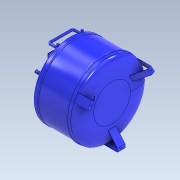
# Autodesk Inventor part: estanque
Saved by Autodesk Inventor 2022 (Build 260153000, 153)
## iProperties
Created: 2022-11-16
Part Number: estanque
Material: Generic
Document SubType Name: Modeling
Designer: ferna
Density: 1 g/cm^3
Appearance: Blue - Wall Paint - Glossy
Author: ferna
Autodesk Inventor part; units mm, degrees
ref_plane "YZ Plane" through (0, 0, 0) normal (1, 0, 0) x (0, 1, 0)
ref_plane "XY Plane" through (0, 0, 0) normal (0, 0, 1) x (1, 0, 0)
sketch "Sketch1" plane through (0, 0, 0) normal (0, 1, 0) x (-1, 0, 0)
  line L0 (0, 0) -> (0, -200)
  line L1 (0, -200) -> (150, -200)
  arc A0 (150, -200) -> (158, -200) centre (154, -197) ccw
  arc A1 (-8, -199.9777) -> (0, -200) centre (-4, -200) ccw
  line L2 (158, -200) -> (173, -200)
  line L3 (-8, -200) -> (-23, -200)
  ellipse E0 centre (173, -100) end of major axis (197.5923, -100) minor radius 100
  line L4 (197.5923, -100) -> (197.5923, 0)
  ellipse E1 centre (-25, -100) end of major axis (-0.4078, -100) minor radius 100
  line L5 (-0.4078, -100) -> (-0.4078, 0)
  line L6 (-49.5923, -100) -> (-49.5923, 0)
  line L7 (-49.5923, 0) -> (197.5923, 0)
  line L8 (-23, -200) -> (-25, -200)
  line L9 (-25, 0) -> (-0.4078, 0)
  point P0 (-25, -200)
  dimension "d0" = 200
  dimension "d1" = 150
  dimension "d2" = 8
  dimension "d3" = 5
  dimension "d4" = 8
  dimension "d5" = 15
  dimension "d6" = 15
  constraints: 20 end point, 7 vertical, 5 horizontal, 5 point on circle, 2 centre point, 1 collinear, 1 perpendicular, 1 point on line, 1 tangent, 10 other
  measures "d0" distance of L0.start L0.end
  measures "d1" distance of L0.end L1.end
  measures "d2" distance of L1.end L2.start
  measures "d3" radius of A0
  measures "d4" distance of L0.end A1.start
  measures "d5" distance of L2.start L2.end
  measures "d6" distance of L3.start L3.end
revolve "Revolution1" add sketch "Sketch1" angle 360 about axis through (49.5923, 0, 0) along (-1, 0, 0)
sketch "Sketch2" plane through (-197.5923, 0, 0) normal (-1, 0, 0) x (0, 0, 1)
  point P0 (0, 0)
ref_plane "Work Plane2" through (0, 189.25, 0) normal (0, 1, 0) x (-1, 0, 0)
sketch "Sketch3" plane through (0, 189.25, 0) normal (0, 1, 0) x (-1, 0, 0)
  circle A0 centre (183.8309, 60.3098) radius 6.2779
  point P0 (0, 0)
  constraints: 1 centre point
sketch3d "3D Sketch1"
  line L0 (-183.8309, 189.25, 60.3098) -> (-183.8309, 179.25, 60.3098)
  arc A0 (-183.8309, 179.25, 60.3098) -> (-193.8309, 169.25, 60.3098) centre (-193.8309, 179.25, 60.3098) ccw
  line L1 (-193.8309, 169.25, 60.3098) -> (-223.8309, 169.25, 60.3098)
  arc A1 (-223.8309, 169.25, 60.3098) -> (-233.8309, 169.25, 50.3098) centre (-223.8309, 169.25, 50.3098) ccw
  line L2 (-233.8309, 169.25, 50.3098) -> (-233.8309, 169.25, -60.7848)
  arc A2 (-233.8309, 169.25, -60.7848) -> (-223.8309, 169.25, -70.7848) centre (-223.8309, 169.25, -60.7848) ccw
  line L3 (-223.8309, 169.25, -70.7848) -> (-193.8309, 169.25, -70.7848)
  arc A3 (-193.8309, 169.25, -70.7848) -> (-183.8309, 179.25, -70.7848) centre (-193.8309, 179.25, -70.7848) ccw
  line L4 (-183.8309, 179.25, -70.7848) -> (-183.8309, 189.25, -70.7848)
  dimension "d9" = 20
  dimension "d10" = 50
  dimension "d11" = 50
  dimension "d12" = 20
  dimension "d13" = 10
  dimension "d14" = 10
  dimension "d15" = 10
  dimension "d16" = 10
sweep "Sweep1" add profiles "Sketch3" path "3D Sketch1"
mirror "Mirror1" about plane through (0, 0, 0) normal (0, 1, 0) of "Sweep1"
ref_plane "Work Plane3" through (99.5923, 0, 0) normal (1, 0, 0) x (0, 0, -1)
sketch "Sketch4" plane through (99.5923, 0, 0) normal (1, 0, 0) x (0, 0, -1)
  circle A0 centre (0, 0) radius 200 projected
  line L0 (21.7689, -198.8118) -> (-20.4699, -198.8118)
  line L1 (-20.4699, -198.8118) -> (-20.4699, -195.5552)
  line L2 (-20.4699, -195.5552) -> (21.7689, -195.5552)
  line L3 (21.7689, -195.5552) -> (21.7689, -198.8118)
  circle A1 centre (0, 0) radius 200 projected
  line L4 (161.2916, 118.2583) -> (182.411, 81.6785)
  line L5 (158.4713, 116.63) -> (161.2916, 118.2583)
  line L6 (179.5907, 80.0502) -> (158.4713, 116.63)
  line L7 (182.411, 81.6785) -> (179.5907, 80.0502)
  line L8 (-183.0605, 80.5534) -> (-161.9411, 117.1333)
  line L9 (-180.2402, 78.9251) -> (-183.0605, 80.5534)
  line L10 (-159.1208, 115.505) -> (-180.2402, 78.9251)
  line L11 (-161.9411, 117.1333) -> (-159.1208, 115.505)
  point P0 (0, 0)
  point P1 (200, 0)
  dimension "d22" = 360
  constraints: 24 end point, 2 parallel, 1 horizontal, 1 perpendicular, 1 point on circle, 25 other
extrude "Extrusion1" add sketch "Sketch4" against normal up to next contours L4 L7 L6 L5 | L8 L11 L10 L9 | L0 L1 L2 L3
sketch "Sketch6" plane through (25, 118.2583, -161.2916) normal (0, 0.8660254, 0.5) x (1, 0, 0)
  line L0 (74.5923, -3.0263) -> (72.0923, -3.0263)
  line L1 (72.0923, -3.0263) -> (72.0923, -18.0263)
  line L2 (72.0923, -18.0263) -> (74.5923, -18.0263)
  line L3 (74.5923, -18.0263) -> (74.5923, -3.0263)
  line L4 (74.5923, -18.0263) -> (-2.5422, -109.9517)
  line L5 (74.5923, -18.0263) -> (194.5923, -18.0263) construction
  line L6 (72.0923, -18.0263) -> (-5.0422, -109.9517)
  line L7 (72.0923, -18.0263) -> (192.0923, -18.0263) construction
  line L8 (-17, -398.8118) -> (-17, 1.1882) projected
  line L9 (-5.0422, -109.9517) -> (-2.5422, -109.9517)
  point P0 (-25, -198.8118)
  dimension "d26" = 2.5
  dimension "d27" = 15
  dimension "d28" = 120
  dimension "d29" = 130
  dimension "d30" = 120
  dimension "d31" = 130
  constraints: 18 end point, 3 horizontal, 2 equal length, 2 parallel, 1 perpendicular
  measures "d26" distance of L2.end L1.end
  measures "d27" distance of L1.end L0.end
  measures "d28" distance of L2.end L4.end
  measures "d29" angle of L4 L5
  measures "d30" distance of L1.end L6.end
  measures "d31" angle of L6 L7
extrude "Extrusion2" add sketch "Sketch6" against normal up to surface (42.2388 mm away)
sketch "Sketch7" plane through (99.5923, -198.8118, 20.4699) normal (0, 0, 1) x (1, 0, 0)
  line L0 (0, 0) -> (0, 3.2566) projected
  line L1 (0, 3.2566) -> (-2.5, 3.2566)
  line L2 (-2.5, 3.2566) -> (-2.5, 18.2566)
  line L3 (-2.5, 18.2566) -> (0, 18.2566)
  line L4 (0, 18.2566) -> (0, 3.2566)
  line L5 (0, 18.2566) -> (-77.1345, 110.1819)
  line L6 (0, 18.2566) -> (120, 18.2566) construction
  line L7 (-2.5, 18.2566) -> (-79.6345, 110.1819)
  line L8 (-2.5, 18.2566) -> (117.5, 18.2566) construction
  line L9 (-79.6345, 110.1819) -> (-77.1345, 110.1819)
  point P0 (-99.5923, 198.8118)
  dimension "d34" = 2.5
  dimension "d35" = 15
  dimension "d36" = 120
  dimension "d37" = 130
  dimension "d38" = 120
  dimension "d39" = 130
  constraints: 18 end point, 3 horizontal, 2 equal length, 2 parallel, 1 perpendicular
  measures "d34" distance of L2.end L3.end
  measures "d35" distance of L1.end L2.end
  measures "d36" distance of L3.end L5.end
  measures "d37" angle of L6 L5
  measures "d38" distance of L2.end L7.end
  measures "d39" angle of L8 L7
extrude "Extrusion3" add sketch "Sketch7" against normal up to surface (42.2388 mm away)
sketch "Sketch8" plane through (25, 80.5534, 183.0605) normal (0, -0.8660254, 0.5) x (1, 0, 0)
  line L0 (74.5923, 0) -> (74.5923, -3.2566) projected
  line L1 (74.5923, -3.2566) -> (72.0923, -3.2566)
  line L2 (72.0923, -3.2566) -> (72.0923, -18.2566)
  line L3 (72.0923, -18.2566) -> (74.5923, -18.2566)
  line L4 (74.5923, -18.2566) -> (74.5923, -3.2566)
  line L5 (74.5923, -18.2566) -> (-2.5422, -110.1819)
  line L6 (74.5923, -18.2566) -> (194.5923, -18.2566) construction
  line L7 (72.0923, -18.2566) -> (-5.0422, -110.1819)
  line L8 (72.0923, -18.2566) -> (192.0923, -18.2566) construction
  line L9 (-25, -398.8118) -> (-25, 1.1882) projected
  line L10 (-5.0422, -110.1819) -> (-2.5422, -110.1819)
  point P0 (-25, -198.8118)
  dimension "d42" = 2.5
  dimension "d43" = 15
  dimension "d44" = 120
  dimension "d45" = 130
  dimension "d46" = 120
  dimension "d47" = 130
  constraints: 18 end point, 3 horizontal, 2 equal length, 2 parallel, 1 perpendicular
  measures "d42" distance of L3.end L2.end
  measures "d43" distance of L2.end L1.end
  measures "d44" distance of L3.end L5.end
  measures "d45" angle of L5 L6
  measures "d46" distance of L2.end L7.end
  measures "d47" angle of L7 L8
extrude "Extrusion4" add sketch "Sketch8" against normal up to surface (42.2388 mm away)
sketch "Sketch9" plane through (99.5923, 0, 0) normal (1, 0, 0) x (0, 0, -1)
  line L0 (-20.4699, -198.8118) -> (21.7689, -198.8118) projected
  line L1 (21.7689, -198.8118) -> (0.6494, -198.8118)
  line L2 (0.6494, -198.8118) -> (0.6494, -189.6833)
  circle A0 centre (0.6494, -189.6833) radius 2.5
  circle A1 centre (163.9458, 95.404) radius 2.5
  circle A2 centre (-164.5952, 94.2792) radius 2.5
  point P0 (0, 0)
  point P1 (0, 0)
  point P2 (0, 0)
  dimension "d50" = 21.1195
  dimension "d51" = 9.1285
  dimension "d52" = 5
  dimension "d55" = 360
  constraints: 4 end point, 3 centre point, 3 coincident, 1 perpendicular, 1 point on line, 8 other
  measures "d50" distance of L0.end L1.end
  measures "d51" distance of L1.end L2.end
  measures "d52" diameter of A0
extrude "Extrusion5" cut sketch "Sketch9" against normal blind 10
sketch "Sketch10" plane through (-197.5923, 0, 0) normal (-1, 0, 0) x (0, 0, 1)
  line L0 (125.5067, 66.7791) -> (-125.5067, 66.7791)
  line L1 (-125.5067, 66.7791) -> (-125.5067, -66.7791)
  line L2 (-125.5067, -66.7791) -> (125.5067, -66.7791)
  line L3 (125.5067, -66.7791) -> (125.5067, 66.7791)
  line L4 (125.5067, 66.7791) -> (-125.5067, -66.7791) construction
  line L5 (-125.5067, 66.7791) -> (125.5067, -66.7791) construction
  circle A0 centre (125.5067, 66.7791) radius 8
  circle A1 centre (125.5067, -66.7791) radius 8
  circle A2 centre (-125.5067, 66.7791) radius 8
  circle A3 centre (-125.5067, -66.7791) radius 8
  line L6 (-60.3098, 136.1742) -> (60.3098, 136.1742)
  line L7 (60.3098, 136.1742) -> (60.3098, -136.1742)
  line L8 (60.3098, -136.1742) -> (-60.3098, -136.1742)
  line L9 (-60.3098, -136.1742) -> (-60.3098, 136.1742)
  line L10 (-60.3098, 136.1742) -> (60.3098, -136.1742) construction
  line L11 (60.3098, 136.1742) -> (-60.3098, -136.1742) construction
  line L12 (-60.3098, 88.4499) -> (60.3098, 88.4499)
  line L13 (60.3098, 88.4499) -> (60.3098, -88.4499)
  line L14 (60.3098, -88.4499) -> (-60.3098, -88.4499)
  line L15 (-60.3098, -88.4499) -> (-60.3098, 88.4499)
  line L16 (-60.3098, 88.4499) -> (60.3098, -88.4499) construction
  line L17 (60.3098, 88.4499) -> (-60.3098, -88.4499) construction
  line L18 (-60.3098, 93.5116) -> (60.3098, 93.5116)
  line L19 (60.3098, 93.5116) -> (60.3098, -93.5116)
  line L20 (60.3098, -93.5116) -> (-60.3098, -93.5116)
  line L21 (-60.3098, -93.5116) -> (-60.3098, 93.5116)
  circle A4 centre (0, 0) radius 100 projected
  line L22 (-60.3098, 93.5116) -> (60.3098, -93.5116) construction
  line L23 (60.3098, 93.5116) -> (-60.3098, -93.5116) construction
  line L24 (-60.3098, 90.6457) -> (60.3098, 90.6457)
  line L25 (60.3098, 90.6457) -> (60.3098, -90.6457)
  line L26 (60.3098, -90.6457) -> (-60.3098, -90.6457)
  line L27 (-60.3098, -90.6457) -> (-60.3098, 90.6457)
  line L28 (-60.3098, 90.6457) -> (60.3098, -90.6457) construction
  line L29 (60.3098, 90.6457) -> (-60.3098, -90.6457) construction
  point P0 (0, 0)
  point P1 (-100, 0)
  dimension "d22" = 360
  dimension "d59" = 16
  dimension "d60" = 16
  dimension "d61" = 16
  dimension "d62" = 16
  constraints: 60 end point, 10 midpoint, 10 parallel, 5 horizontal, 5 perpendicular, 4 centre point, 4 coincident, 3 point on line, 1 horizontal alignment
  measures "d59" diameter of A0
  measures "d60" diameter of A1
  measures "d61" diameter of A2
  measures "d62" diameter of A3
extrude "Extrusion6" add sketch "Sketch10" along normal blind 40 and the other way blind 25.375 contours A2 L1 L0 | L0 L1 A2 | A3 L2 L1 | L1 L2 A3 | L9 L24 A4 L12 | A4 L24 L12 | A4 L24 L7 L12 | L14 A4 L26 L9 | L14 A4 L26 | A0 L3 L0 | L0 L3 A0 | L14 L7 L26 A4 | A1 L3 L2 | L2 L3 A1
sketch "Sketch11" plane through (-237.5923, 0, 0) normal (-1, 0, 0) x (0, 0, 1)
  line L0 (-60.3098, 88.4499) -> (60.3098, 88.4499)
  line L1 (60.3098, 88.4499) -> (60.3098, 118.4499)
  line L2 (60.3098, 118.4499) -> (-60.3098, 118.4499)
  line L3 (-60.3098, 118.4499) -> (-60.3098, 88.4499)
  line L4 (60.3098, -88.4499) -> (-60.3098, -88.4499) projected
  line L5 (-60.3098, -88.4499) -> (60.3098, -88.4499)
  line L6 (60.3098, -88.4499) -> (60.3098, -118.4499)
  line L7 (60.3098, -118.4499) -> (-60.3098, -118.4499)
  line L8 (-60.3098, -118.4499) -> (-60.3098, -88.4499)
  line L9 (-50, -105) -> (50, -105)
  line L10 (50, -105) -> (50, 105)
  line L11 (50, 105) -> (-50, 105)
  line L12 (-50, 105) -> (-50, -105)
  line L13 (-50, -105) -> (50, 105) construction
  line L14 (50, -105) -> (-50, 105) construction
  circle A0 centre (-50, 105) radius 5
  circle A1 centre (50, 105) radius 5
  circle A2 centre (-50, -105) radius 5
  circle A3 centre (50, -105) radius 5
  point P0 (0, 0)
  dimension "d67" = 30
  dimension "d68" = 30
  dimension "d69" = 100
  dimension "d70" = 210
  dimension "d71" = 10
  dimension "d72" = 10
  dimension "d73" = 10
  dimension "d74" = 10
  constraints: 28 end point, 6 parallel, 4 centre point, 4 coincident, 3 horizontal, 3 perpendicular, 2 midpoint, 1 point on line
  measures "d67" distance of L1.end L0.end
  measures "d68" distance of L5.end L6.end
  measures "d69" distance of L11.end L10.end
  measures "d70" distance of L10.end L9.end
  measures "d71" diameter of A0
  measures "d72" diameter of A1
  measures "d73" diameter of A2
  measures "d74" diameter of A3
extrude "Extrusion7" add sketch "Sketch11" along normal blind 1.5 contours L3 L2 L1 L0 L10 A1 L11 A0 L12 | L12 A0 L11 A1 L10 L0 | L12 A2 L9 A3 L10 L4 L6 L7 L8 | L4 L10 A3 L9 A2 L12
equation "\"d14\" = d13"
equation "\"d15\" = d13"
equation "\"d16\" = d13"
body "Solid1"
